pully 2GT-10mm 8mm v3 (Autodesk Fusion 360 design; units mm, degrees)
Autodesk Fusion 360 part; units mm, degrees
sketch "Sketch1" plane through (0, 0, 0) normal (0, 0, 1) x (1, 0, 0)
  circle A0 centre (0, 0) radius 8
  circle A1 centre (0, 0) radius 4
  dimension "d1" = 16
  dimension "d2" = 8
  constraint coincident A0.centre A1.centre
  measures "d1" diameter of A0
  measures "d2" diameter of A1
extrude "Extrude1" add sketch "Sketch1" along normal blind 7.6
sketch "Sketch2" plane through (0, 0, 7.6) normal (0, 0, 1) x (-1, 0, 0)
  circle A0 centre (0, 0) radius 4
  circle A1 centre (0, 0) radius 8
  circle A2 centre (0, 0) radius 6
  dimension "d5" = 12
  constraint coincident A0.centre A1.centre
  measures "d5" diameter of A2
extrude "Extrude2" add sketch "Sketch2" along normal blind 11 contours A2
sketch "Sketch3" plane through (0, 0, 18.6) normal (0, 0, 1) x (-1, 0, 0)
  circle A0 centre (0, 0) radius 4
  circle A1 centre (0, 0) radius 6
  circle A2 centre (0, 0) radius 8
  dimension "d8" = 16
  constraint coincident A0.centre A1.centre
  measures "d8" diameter of A2
extrude "Extrude3" add sketch "Sketch3" along normal blind 1.2 contours A1 | A2
